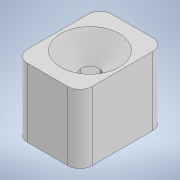
# Autodesk Inventor part: 센서부 90
Saved by Autodesk Inventor 2022 (Build 260153000, 153)
## iProperties
Created: 2023-11-20
Part Number: 센서부 90
Material: 일반
Document SubType Name: Modeling
Designer: USER
Density: 1 g/cm^3
Appearance: 기본값
Author: USER
Autodesk Inventor part; units mm, degrees
ref_plane "YZ Plane" through (0, 0, 0) normal (1, 0, 0) x (0, 1, 0)
ref_plane "XZ Plane" through (0, 0, 0) normal (0, 1, 0) x (-1, 0, 0)
ref_plane "XY Plane" through (0, 0, 0) normal (0, 0, 1) x (1, 0, 0)
sketch "스케치1" plane through (0, 0, 0) normal (0, 1, 0) x (-1, 0, 0)
  line L0 (-3.5031, -21.0217) -> (-3.5031, -19.0217)
  line L1 (-2.5031, -19.0217) -> (-2.5031, -16.0217)
  line L2 (-2.0031, -16.5217) -> (-0.0031, -16.5217)
  line L3 (-12.5031, -19.0217) -> (-12.5031, -21.0217)
  line L4 (-13.5031, -16.0217) -> (-13.5031, -19.0217)
  line L5 (-13.5031, -19.0217) -> (-2.5031, -19.0217)
  line L6 (-2.5031, -16.0217) -> (-13.5031, -16.0217)
  line L7 (-14.0031, -19.0217) -> (-2.0031, -19.0217)
  line L8 (-16.0031, -16.5217) -> (-14.0031, -16.5217)
  line L9 (-0.0031, -21.0217) -> (-16.0031, -21.0217)
  circle A0 centre (-8.0031, -10.5217) radius 5
  line L10 (-0.0031, -21.0217) -> (-0.0031, -0.0217)
  line L11 (-16.0031, -21.0217) -> (-16.0031, -0.0217)
  circle A1 centre (-8.0031, -10.5217) radius 7
  line L12 (-14.0031, -2.0217) -> (-14.0031, -19.0217)
  line L13 (-2.0031, -19.0217) -> (-2.0031, -2.0217)
  line L14 (-2.0031, -4.5217) -> (-0.0031, -4.5217)
  line L15 (-3.5031, -2.0217) -> (-3.5031, -0.0217)
  line L16 (-12.5031, -2.0217) -> (-12.5031, -0.0217)
  line L17 (-14.0031, -4.5217) -> (-16.0031, -4.5217)
  line L18 (-2.0031, -2.0217) -> (-14.0031, -2.0217)
  line L19 (-16.0031, -0.0217) -> (-0.0031, -0.0217)
  circle A2 centre (-8.0031, -10.5217) radius 2.25
  point P0 (0, 0)
  point P1 (-2.0031, -6.9161)
  point P2 (-2.0031, -14.1272)
  point P3 (-14.0031, -14.1272)
  point P4 (-14.0031, -6.9161)
  dimension "d0" = 21
  dimension "d1" = 4.5
  dimension "d19" = 17
  dimension "d20" = 12
  dimension "d21" = 10
  constraints: 40 end point, 3 centre point, 1 coincident
  measures "d0" distance between parallel lines of L9 L19
  measures "d1" diameter of A2
  measures "d19" distance of L18.end L12.end
  measures "d20" distance of L18.start L18.end
  measures "d21" diameter of A0
extrude "돌출2" add sketch "스케치1" against normal blind 12 contours L9 L3 L5 L0 | L0 L5 L7 L13 L2 L10 L9 | L9 L11 L8 L12 L7 L5 L3 | L2 L13 A1 L14 L10 | L14 L13 L18 L15 L19 L10 | L11 L17 L12 A1 L8 | L11 L19 L16 L18 L12 L17 | L15 L18 L16 L19
extrude "돌출3" add sketch "스케치1" along normal blind 5 contours L9 L3 L5 L0 | L0 L5 L7 L13 L2 L10 L9 | L5 L4 L6 A1 L1 | L9 L11 L8 L12 L7 L5 L3 | L1 L6 A1 L13 L7 | L2 L13 A1 L14 L10 | L7 L12 A1 L6 L4 | L14 L13 L18 L15 L19 L10 | L11 L17 L12 A1 L8 | A1 L6 | L6 A1 L12 L13 | L13 A1 | L13 A1 L12 L18 | L11 L19 L16 L18 L12 L17 | L15 L18 L16 L19 | A1 L12 | A0 | A2
extrude "돌출4" cut sketch "스케치1" along normal blind 13 contours A2
sketch "스케치2" plane through (0, 5, 0) normal (0, 1, 0) x (1, 0, 0)
  point P0 (0, 0)
  point P1 (8.0031, 10.5217)
sketch "스케치3" plane through (0, 5, 0) normal (0, 1, 0) x (1, 0, 0)
  circle A0 centre (8.0031, 10.5217) radius 2.25 projected
  circle A1 centre (8.0031, 10.5217) radius 5
  point P0 (0, 0)
  dimension "d10" = 10
  constraints: 1 centre point, 1 coincident
  measures "d10" diameter of A1
fillet "모깎기1" radius 3 4 edges at (16.0031, -3.5, -21.0217) (0.0031, -3.5, -21.0217) (16.0031, -3.5, -0.0217) (0.0031, -3.5, -0.0217)
chamfer "모따기1" distance 5 angle 45 1 edges at (10.2531, 5, -10.5217) measured on face at (1.9198, 5, -10.5217)
